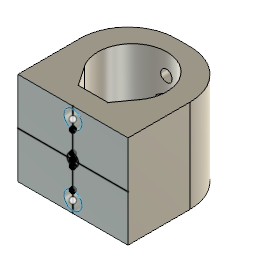
penplotter v3 (Autodesk Fusion 360 design; units mm, degrees)
Autodesk Fusion 360 part; units mm, degrees
sketch "スケッチ1" plane through (0, 0, 0) normal (0, 0, 1) x (1, 0, 0)
  line L0 (0, 0) -> (32, 0)
  line L1 (32, 0) -> (32, 32)
  line L2 (32, 32) -> (0, 32)
  line L3 (0, 32) -> (0, 0)
  dimension "d1" = 32
  dimension "d2" = 32
  constraint horizontal L0
  constraint vertical L1
  constraint horizontal L2
  constraint vertical L3
  constraint coincident L0.start L3.end
  measures "d1" distance of L0.start L0.end
  measures "d2" distance of L0.start L2.end
extrude "押し出し1" add sketch "スケッチ1" along normal blind 27
sketch "スケッチ2" plane through (0, 0, 0) normal (0, -1, 0) x (1, 0, 0)
  line L0 (0, 0) -> (32, 0)
  line L1 (32, 0) -> (32, 27)
  line L2 (32, 27) -> (0, 27)
  line L3 (0, 27) -> (0, 0)
  line L4 (16, 27) -> (16, 0)
  line L5 (0, 13.5) -> (32, 13.5)
  circle A0 centre (16, 13.5) radius 1.6
  circle A1 centre (15.9997, 23.7) radius 2.6
  circle A2 centre (16.0002, 3.3) radius 2.6
  point P0 (16, 21.1)
  point P1 (16, 5.9)
  point P2 (16, 15.1)
  point P3 (16, 11.9)
  dimension "d5" = 3.2
  dimension "d18" = 5.2
  dimension "d19" = 5.2
  dimension "d27" = 6
  dimension "d28" = 6
  constraint midpoint L2 L4.start
  constraint midpoint L0 L4.end
  constraint midpoint L3 L5.start
  constraint midpoint L1 L5.end
  constraint midpoint L5 A0.centre
  constraint coincident L4 P0
  constraint coincident L4 P1
  constraint coincident P0 A1
  constraint coincident P1 A2
  constraint coincident A0 P2
  constraint coincident L4 P2
  constraint coincident L4 P3
  constraint coincident A0 P3
  measures "d5" diameter of A0
  measures "d18" diameter of A2
  measures "d19" diameter of A1
  measures "d27" distance of P0 P2
  measures "d28" distance of P1 P3
sketch "スケッチ3" plane through (0, 0, 27) normal (0, 0, 1) x (-1, 0, 0)
  line L0 (0, -32) -> (0, 0)
  line L1 (0, 0) -> (-32, 0)
  line L2 (-32, 0) -> (-32, -32)
  line L3 (-32, -32) -> (0, -32)
  line L4 (0, -25) -> (-32, -25)
  circle A0 centre (-16, -17.25) radius 10
  line L5 (-16, -25) -> (-16, -6)
  line L6 (-16, -6) -> (-11.5866, -6)
  line L7 (-16, -6) -> (-20.1944, -6)
  line L8 (-11.5866, -6) -> (-7.751, -11.5972)
  line L9 (-20.1944, -6) -> (-24.0954, -11.3793)
  dimension "d6" = 7
  dimension "d7" = 20
  dimension "d20" = 6
  constraint coincident L0 L4.start
  constraint coincident L2 L4.end
  constraint perpendicular L2 L4
  constraint midpoint L4 L5.start
  constraint perpendicular L4 L5
  constraint perpendicular L5 L6
  constraint perpendicular L5 L7
  constraint coincident A0 L8.end
  constraint tangent A0 L8
  constraint coincident A0 L9.end
  constraint tangent A0 L9
  measures "d6" distance of L3 L4
  measures "d7" diameter of A0
  measures "d20" distance of L1 L5.end
extrude "押し出し2" cut sketch "スケッチ3" against normal blind 75 contours L4 A0 | L4 A0 L5 | L4 A0 L5 | A0 L5 L6 L8 | A0 L5 L7 L9
extrude "押し出し3" cut sketch "スケッチ2" against normal blind 15 contours L4 A2 | L4 A2 | L4 L5 A0 | L4 L5 A0 | L4 L5 A0 | L4 L5 A0 | L4 A1 | L4 A1
ref_plane "作業平面1" through (16, 10, 13.5) normal (0, -1, 0) x (1, 0, 0)
sketch "スケッチ4" plane through (0, 10, 0) normal (0, -1, 0) x (-1, 0, 0)
sketch "スケッチ5" plane through (0, 10, 0) normal (0, -1, 0) x (-1, 0, 0)
  circle A0 centre (-16, -13.5) radius 2.9
  dimension "d13" = 5.8
  measures "d13" diameter of A0
extrude "押し出し4" cut sketch "スケッチ5" along normal blind 7
sketch "スケッチ6" plane through (0, 32, 0) normal (0, 1, 0) x (-1, 0, 0)
  line L0 (-32, 0) -> (0, 0)
  line L1 (0, 0) -> (0, 27)
  line L2 (0, 27) -> (-32, 27)
  line L3 (-32, 27) -> (-32, 0)
  line L4 (-16, 27) -> (-16, 0)
  line L5 (-32, 13.5) -> (0, 13.5)
  circle A0 centre (-16, 13.5) radius 1.65
  circle A1 centre (-16, 21) radius 1.65
  circle A2 centre (-16, 6) radius 1.65
  dimension "d21" = 3.3
  dimension "d22" = 3.3
  dimension "d23" = 3.3
  constraint midpoint L2 L4.start
  constraint midpoint L0 L4.end
  constraint midpoint L3 L5.start
  constraint midpoint L1 L5.end
  constraint midpoint L5 A0.centre
  constraint coincident L4 A1.centre
  constraint coincident L4 A2.centre
  measures "d21" diameter of A0
  measures "d22" diameter of A1
  measures "d23" diameter of A2
extrude "押し出し5" cut sketch "スケッチ6" against normal blind 10 contours L4 A2 | L4 A2 | L4 L5 A0 | L4 L5 A0 | L4 L5 A0 | L4 L5 A0 | L4 A1 | L4 A1
ref_plane "作業平面2" through (16, 25, 13.5) normal (0, 1, 0) x (-1, 0, 0)
sketch "スケッチ7" plane through (0, 25, 0) normal (0, 1, 0) x (1, 0, 0)
  line L0 (13.25, -15.0877) -> (16, -16.6754)
  line L1 (16, -16.6754) -> (18.75, -15.0877)
  line L2 (18.75, -15.0877) -> (18.75, -11.9123)
  line L3 (18.75, -11.9123) -> (16, -10.3246)
  line L4 (16, -10.3246) -> (13.25, -11.9123)
  line L5 (13.25, -11.9123) -> (13.25, -15.0877)
  point P0 (16, -13.5)
  dimension "d30" = 2.75
  measures "d30" distance of P0 L5
extrude "押し出し6" cut sketch "スケッチ7" along normal blind 5
fillet "フィレット1" radius 14 2 edges at (0, 32, 13.5) (32, 32, 13.5)
